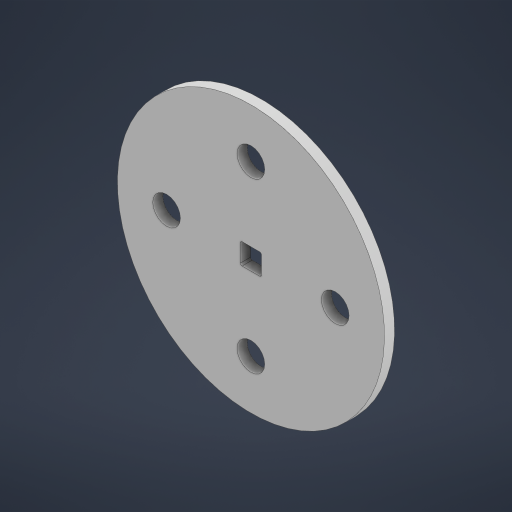
# Autodesk Inventor part: HS adapter retainer
Saved by Autodesk Inventor 2023.2 (Build 272271000, 271)
## iProperties
Created: 2023-03-21
Part Number: HS adapter retainer
Material: Generic
Document SubType Name: Modeling
Designer: Liam
Density: 1 g/cm^3
Appearance: Default
Author: Liam
Autodesk Inventor part; units mm, degrees
ref_plane "YZ Plane" through (0, 0, 0) normal (1, 0, 0) x (0, 1, 0)
ref_plane "XZ Plane" through (0, 0, 0) normal (0, 1, 0) x (-1, 0, 0)
ref_plane "XY Plane" through (0, 0, 0) normal (0, 0, 1) x (1, 0, 0)
sketch "Sketch1" plane through (0, 0, 0) normal (0, 0, 1) x (1, 0, 0)
  circle A0 centre (0, 12.7) radius 2.0828
  circle A1 centre (12.7, 0) radius 2.0828
  circle A2 centre (0, -12.7) radius 2.0828
  circle A3 centre (-12.7, 0) radius 2.0828
  arc A4 (5.5881, 19.3163) -> (4.8187, 19.5224) centre (0, 0) ccw projected
  circle A5 centre (0, 0) radius 20.1083
  line L0 (-1.5875, 1.3335) -> (-1.5875, -1.3335)
  line L1 (-1.3335, -1.5875) -> (1.3335, -1.5875)
  line L2 (1.5875, -1.3335) -> (1.5875, 1.3335)
  arc A6 (1.5875, 1.3335) -> (1.3335, 1.5875) centre (1.3335, 1.3335) ccw
  arc A7 (-1.3335, 1.5875) -> (-1.5875, 1.3335) centre (-1.3335, 1.3335) ccw
  arc A8 (-1.5875, -1.3335) -> (-1.3335, -1.5875) centre (-1.3335, -1.3335) ccw
  arc A9 (1.3335, -1.5875) -> (1.5875, -1.3335) centre (1.3335, -1.3335) ccw
  line L3 (-1.3335, 1.5875) -> (1.3335, 1.5875)
  point P0 (0, 0)
  point P1 (5.5881, 19.3163)
  point P2 (1.5875, 1.5875)
  point P3 (1.5875, 0)
  point P4 (0, -1.5875)
  point P5 (0, 1.5875)
  point P6 (4.8187, 19.5224)
  dimension "halfLength" = 1.5875
  dimension "d16" = 1.5875
  dimension "d17" = 1.5875
  dimension "d18" = 1.5875
  dimension "d20" = 0.254
  dimension "d21" = 2.667
  dimension "d22" = 2.667
  dimension "d23" = 40.2167
  dimension "d24" = 4.1656
  dimension "d25" = 4.1656
  dimension "d26" = 4.1656
  dimension "d27" = 4.1656
  constraints: 9 centre point, 8 end point, 8 point on circle, 6 tangent, 3 equal radius, 3 midpoint, 3 perpendicular, 1 coincident, 1 point on line, 1 vertical, 4 other
  measures "halfLength" distance from line of L3 point (0, 0)
  measures "d16" distance from line of L1 point (0, 0)
  measures "d17" distance from line of L2 point (0, 0)
  measures "d18" distance from line of L0 A4.centre
  measures "d20" radius of A6
  measures "d21" distance of L0.start L0.end
  measures "d22" distance of L3.start L3.end
  measures "d23" diameter of A5
  measures "d24" diameter of A0
  measures "d25" diameter of A3
  measures "d26" diameter of A2
  measures "d27" diameter of A1
extrude "Extrusion3" add sketch "Sketch1" along normal blind 1.524
equation "\"d16\" = halfLength"
equation "\"d17\" = halfLength"
equation "\"d18\" = d17"
equation "\"d21\" = 2 * halfLength - 2 * d20"
equation "\"d22\" = d21"
equation "\"d25\" = d24"
equation "\"d26\" = d24"
equation "\"d27\" = d24"
body "Solid3"
